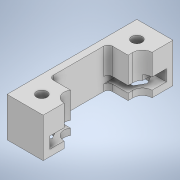
# Autodesk Inventor part: krepl_1.2
Saved by Autodesk Inventor 2021.1 (Build 251245010, 245A)
## iProperties
Created: 2023-04-14
Part Number: krepl_1.2
Material: Типовые
Document SubType Name: Modeling
Designer: User
Density: 1 g/cm^3
Appearance: По умолчанию
Author: User
Autodesk Inventor part; units mm, degrees
ref_plane "YZ Plane" through (0, 0, 0) normal (1, 0, 0) x (0, 1, 0)
ref_plane "XZ Plane" through (0, 0, 0) normal (0, 1, 0) x (-1, 0, 0)
ref_plane "XY Plane" through (0, 0, 0) normal (0, 0, 1) x (1, 0, 0)
sketch "Эскиз1" plane through (0, 0, 0) normal (0, 1, 0) x (-1, 0, 0)
  line L0 (0, 0) -> (9, 0)
  line L1 (9, 0) -> (9, -35.56)
  line L2 (9, -35.56) -> (0, -35.56)
  line L3 (0, -35.56) -> (0, 0)
  line L4 (-8.5, -9.28) -> (7.5, -9.28)
  line L5 (8.5, -10.28) -> (8.5, -25.28)
  line L6 (7.5, -26.28) -> (-8.5, -26.28)
  line L7 (-8.5, -26.28) -> (-8.5, -9.28)
  line L8 (-8.5, -9.28) -> (8.5, -26.28) construction
  line L9 (8.5, -9.28) -> (-8.5, -26.28) construction
  circle A0 centre (7.5, -10.28) radius 1
  circle A1 centre (7.5, -25.28) radius 1
  line L10 (7.5, -9.28) -> (8.5, -9.28) construction
  line L11 (8.5, -10.28) -> (8.5, -9.28) construction
  line L12 (7.5, -26.28) -> (8.5, -26.28) construction
  line L13 (8.5, -26.28) -> (8.5, -25.28) construction
  line L14 (9, -25.28) -> (9, -10.28)
  line L15 (9, -10.28) -> (9, -8.78)
  line L16 (9, -8.78) -> (7.5, -8.78)
  line L17 (7.5, -8.78) -> (-9, -8.78)
  line L18 (-9, -8.78) -> (-9, -26.78)
  line L19 (-9, -26.78) -> (7.5, -26.78)
  line L20 (7.5, -26.78) -> (9, -26.78)
  line L21 (9, -26.78) -> (9, -25.28)
  line L22 (11, 2) -> (-2, 2)
  line L23 (-2, 2) -> (-2, -37.56)
  line L24 (-2, -37.56) -> (11, -37.56)
  line L25 (11, -37.56) -> (11, 2)
  line L26 (0, 2) -> (0, 0)
  line L27 (0, -35.56) -> (0, -37.56)
  circle A2 centre (5.7, -32.26) radius 1.6
  line L28 (0, -17.78) -> (11, -17.78) construction
  circle A3 centre (5.7, -3.3) radius 1.6
  point P0 (0, -26.78)
  point P1 (0, -8.78)
  dimension "d0" = 17
  dimension "d1" = 17
  dimension "d2" = 35.56
  dimension "d3" = 2
  dimension "d4" = 90
  dimension "d5" = 0.5
  dimension "d6" = 2
  dimension "d7" = 3.2
  dimension "d8" = 3.3
  dimension "d9" = 3.3
  constraints: 58 end point, 8 parallel, 8 perpendicular, 6 point on line, 4 centre point, 4 midpoint, 4 point on circle, 3 horizontal, 3 tangent, 1 collinear, 1 equal radius, 1 symmetric about line, 1 vertical, 11 other
  measures "d0" distance of L8.end L6.end
  measures "d1" distance of L9.start L8.end
  measures "d2" distance of L0.end L1.end
  measures "d3" diameter of A0
  measures "d4" angle of L8 L9
  measures "d5" distance between parallel lines of L14 L5
  measures "d6" distance between parallel lines of L25 L1
  measures "d7" diameter of A2
  measures "d8" distance from line of L1 A2.centre
  measures "d9" distance from line of L2 A2.centre
extrude "Выдавливание1" add sketch "Эскиз1" along normal blind 12 contours L26 L22 L25 L24 L27 L2 L1 L0 | L0 L1 L16 L17 L3 | L19 L20 L1 L2 L3
sketch "Эскиз2" plane through (0, 0, 0) normal (0, -1, 0) x (1, 0, 0)
  circle A0 centre (-5.7, -32.26) radius 1.6 projected
  line L0 (-2.4668, -32.26) -> (-4.0834, -35.06)
  line L1 (-4.0834, -35.06) -> (-7.3166, -35.06)
  line L2 (-7.3166, -35.06) -> (-8.9332, -32.26)
  line L3 (-8.9332, -32.26) -> (-7.3166, -29.46)
  line L4 (-7.3166, -29.46) -> (-4.0834, -29.46)
  line L5 (-4.0834, -29.46) -> (-2.4668, -32.26)
  line L6 (-11, -37.56) -> (-11, 2) projected
  line L7 (-11, -17.78) -> (0, -17.78) construction
  circle A1 centre (-5.7, -3.3) radius 1.6
  line L8 (-2.4668, -3.3) -> (-4.0834, -0.5)
  line L9 (-4.0834, -0.5) -> (-7.3166, -0.5)
  line L10 (-7.3166, -0.5) -> (-8.9332, -3.3)
  line L11 (-8.9332, -3.3) -> (-7.3166, -6.1)
  line L12 (-7.3166, -6.1) -> (-4.0834, -6.1)
  line L13 (-4.0834, -6.1) -> (-2.4668, -3.3)
  point P0 (0, 0)
  dimension "d12" = 5.6
  constraints: 26 end point, 8 symmetric about line, 2 coincident, 2 horizontal, 1 centre point, 1 midpoint, 14 other
  measures "d12" distance between parallel lines of L1 L4
extrude "Выдавливание2" cut sketch "Эскиз2" against normal blind 2 contours L0 L1 L2 L3 L4 L5 | A1 | L13 L12 L11 L10 L9 L8
sketch "Эскиз3" plane through (0, 0, -26.78) normal (1, 0, 0) x (0, 0, -1)
  line L0 (-28.78, 0) -> (-28.78, 12) projected
  line L1 (10.78, 0) -> (-28.78, 0)
  line L2 (-28.78, 0) -> (-28.78, 12)
  line L3 (-28.78, 12) -> (10.78, 12)
  line L4 (10.78, 12) -> (10.78, 0)
  line L5 (8.78, 10) -> (-26.78, 10)
  line L6 (-26.78, 10) -> (-26.78, 2)
  line L7 (-26.78, 2) -> (8.78, 2)
  line L8 (8.78, 2) -> (8.78, 10)
  line L9 (10.78, 0) -> (10.78, 12) projected
  line L10 (-28.78, 0) -> (-18, 0) projected
  line L11 (8.78, 4) -> (-26.78, 4)
  point P0 (-26.78, 0)
  dimension "d15" = 2
  dimension "d16" = 2
  constraints: 18 end point, 4 parallel, 3 perpendicular, 2 collinear, 2 point on line, 1 horizontal, 3 other
  measures "d15" distance between parallel lines of L0 L6
  measures "d16" distance between parallel lines of L7 L11
extrude "Выдавливание3" cut sketch "Эскиз3" against normal up to surface (9 mm away) contours L8 L7 L6 L11
fillet "Сопряжение1" radius 1.3 4 edges at (-9, 1, -8.78) (-9, 8, -8.78) (-9, 1, -26.78) (-9, 8, -26.78)
sketch "Эскиз4" plane through (0, 12, 0) normal (0, 1, 0) x (1, 0, 0)
  line L0 (-7.7, 26.78) -> (0, 26.78) projected
  line L1 (-2.4, 26.78) -> (2.4, 26.78)
  line L2 (2.4, 26.78) -> (2.4, 28.28)
  line L3 (2.4, 28.28) -> (-2.4, 28.28)
  line L4 (-2.4, 28.28) -> (-2.4, 26.78)
  line L5 (0, 26.78) -> (-2.4, 28.28) construction
  line L6 (2.4, 28.28) -> (0, 26.78) construction
  line L7 (0, 26.78) -> (0, 37.56) projected
  circle A0 centre (0, 28.28) radius 2.4
  line L8 (0, 17.78) -> (-11, 17.78) construction
  line L9 (-11, 37.56) -> (-11, -2) projected
  line L10 (-2.4, 8.78) -> (2.4, 8.78)
  line L11 (2.4, 8.78) -> (2.4, 7.28)
  line L12 (2.4, 7.28) -> (-2.4, 7.28)
  line L13 (-2.4, 7.28) -> (-2.4, 8.78)
  line L14 (0, 8.78) -> (-2.4, 7.28) construction
  line L15 (2.4, 7.28) -> (0, 8.78) construction
  circle A1 centre (0, 7.28) radius 2.4
  line L16 (-11, -2) -> (0, 17.78) construction
  line L17 (0, 37.56) -> (-11, 37.56) projected
  line L18 (0, 17.78) -> (-11, 37.56) construction
  line L19 (-2.9, 26.28) -> (2.9, 26.28)
  line L20 (2.9, 26.28) -> (2.9, 28.78)
  line L21 (2.9, 28.78) -> (-2.9, 28.78)
  line L22 (-2.9, 28.78) -> (-2.9, 26.28)
  circle A2 centre (0, 28.28) radius 2.9
  circle A3 centre (0, 7.28) radius 2.9
  line L23 (2.9, 6.78) -> (2.9, 9.28)
  line L24 (2.9, 9.28) -> (-2.9, 9.28)
  line L25 (-2.9, 9.28) -> (-2.9, 6.78)
  line L26 (-2.9, 6.78) -> (2.9, 6.78)
  point P0 (0, 0)
  point P1 (-2.9, 28.28)
  point P2 (-2.9, 26.78)
  point P3 (0, 31.18)
  point P4 (1.8735, 8.78)
  point P5 (1.8735, 8.78)
  point P6 (-1.8735, 8.78)
  point P7 (-1.8735, 8.78)
  point P8 (-1.9, 8.7463)
  point P9 (-2.1, 9.28)
  point P10 (-2.9, 7.28)
  dimension "d20" = 4.8
  dimension "d21" = 1.5
  dimension "d22" = 0.5
  dimension "d23" = 0.5
  constraints: 46 end point, 7 symmetric about line, 5 midpoint, 4 parallel, 4 point on line, 2 centre point, 2 equal length, 2 horizontal, 2 perpendicular, 2 tangent, 1 horizontal alignment, 11 other
  measures "d20" distance between parallel lines of L2 L4
  measures "d21" distance between parallel lines of L3 L1
  measures "d22" distance between parallel lines of L4 L22
  measures "d23" distance between parallel lines of L23 L11
extrude "Выдавливание4" cut sketch "Эскиз4" against normal up to surface (12 mm away) contours L22 A2 L0 | A2 L21 A0 L4 L0 | L4 A0 L0 | A2 L7 A0 L21 | A0 L3 L7 L0 | A0 L21 L7 L3 | A0 L7 L21 | L13 A1 L26 A3 L24 L10 | L10 A1 L13 | A1 L24 L10 | L10 A1 L12 | L12 A1 L26 | A1 L24 A3 L26 L11 L10 | L10 L11 A1 | L24 A3 A1 | A1 L24 | L26 A1 | A1 L26 A3 picked at (-0.403, 30.9667) picked at (-0.7824, 28.6133) picked at (-1.5074, 28.9517)
sketch "Эскиз5" plane through (0, 0, 2) normal (1, 0, 0) x (0, 0, -1)
  line L0 (10.78, 12) -> (10.78, 4) projected
  line L1 (2, 2) -> (2, 4) projected
  line L2 (2, 4) -> (10.78, 4)
  line L3 (10.78, 4) -> (10.78, 5.5)
  line L4 (10.78, 5.5) -> (2, 5.5)
  line L5 (2, 5.5) -> (2, 4)
  line L6 (30.28, 12) -> (30.28, 4) projected
  line L7 (37.56, 4) -> (37.56, 2) projected
  line L8 (33.18, 4) -> (37.56, 4) projected
  line L9 (37.56, 4) -> (30.28, 4)
  line L10 (30.28, 4) -> (30.28, 5.5)
  line L11 (30.28, 5.5) -> (37.56, 5.5)
  line L12 (37.56, 5.5) -> (37.56, 4)
  point P0 (2, 0)
  point P1 (10.78, 4)
  dimension "d26" = 1.5
  constraints: 16 end point, 5 parallel, 2 horizontal, 2 perpendicular, 2 point on line
  measures "d26" distance between parallel lines of L2 L4
extrude "Выдавливание5" cut sketch "Эскиз5" against normal blind 2
